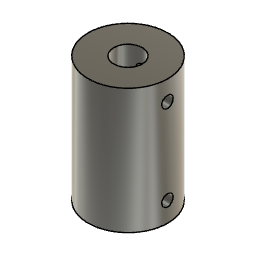
coupling (Autodesk Fusion 360 design; units mm, degrees)
Autodesk Fusion 360 part; units mm, degrees
note: some values were not read from the file. Set by a fixed rule: which sketch regions a step uses.
sketch "スケッチ1" plane through (0, 0, 0) normal (0, 0, 1) x (1, 0, 0)
  circle A0 centre (0, 0) radius 7
  dimension "d1" = 14
  constraint coincident A0.centre origin
  measures "d1" diameter of A0
extrude "押し出し1" add sketch "スケッチ1" along normal blind 12
extrude "押し出し2" add 1 faces at (1.11, -1.8763, 12) along direction (0, 0, 1) blind 10
sketch "スケッチ2" plane through (0, 0, 22) normal (0, 0, 1) x (-1, 0, 0)
  circle A0 centre (0, 0) radius 7
  circle A1 centre (0, 0) radius 2.5
  dimension "d6" = 5
  constraint coincident A0.centre A1.centre
  measures "d6" diameter of A1
sketch "スケッチ3" plane through (0, 0, 0) normal (0, 0, -1) x (1, 0, 0)
  circle A0 centre (0, 0) radius 7
  circle A1 centre (0, 0) radius 1.5
  dimension "d7" = 3
  constraint coincident A0.centre A1.centre
  measures "d7" diameter of A1
extrude "押し出し3" cut sketch "スケッチ3" against normal blind 11 contours A1
extrude "押し出し4" cut sketch "スケッチ2" against normal blind 11 contours A1
sketch "スケッチ4" plane through (0, 0, 0) normal (0, 1, 0) x (1, 0, 0)
  line L0 (-7, -22) -> (7, -22)
  line L1 (7, -22) -> (7, 0)
  line L2 (7, 0) -> (-7, 0)
  line L3 (-7, 0) -> (-7, -22)
  line L4 (-7, -22) -> (-7, -18.5)
  line L5 (-7, -18.5) -> (7, -18.5)
  line L6 (7, -22) -> (7, -18.5)
  line L7 (0, -22) -> (0, 0)
  circle A0 centre (0, -18.5) radius 1
  line L8 (-7, 0) -> (-7, -3.5)
  line L9 (-7, -3.5) -> (7, -3.5)
  circle A1 centre (0, -3.5) radius 1
  dimension "d12" = 3.5
  dimension "d13" = 2
  dimension "d20" = 3.5
  dimension "d21" = 2
  constraint horizontal L0
  constraint vertical L1
  constraint horizontal L2
  constraint vertical L3
  constraint perpendicular L0 L4
  constraint coincident L1 L5.end
  constraint perpendicular L1 L5
  constraint midpoint L0 L7.start
  constraint coincident L7.end origin
  constraint perpendicular L2 L7
  constraint midpoint L5 A0.centre
  constraint perpendicular L2 L8
  constraint coincident L1 L9.end
  constraint perpendicular L1 L9
  constraint midpoint L9 A1.centre
  measures "d12" distance of L0.start L4.end
  measures "d13" diameter of A0
  measures "d20" distance of L2.end L8.end
  measures "d21" diameter of A1
extrude "押し出し5" cut sketch "スケッチ4" along normal blind 10 contours L5 L7 A0 | L5 L7 A0 | L5 L7 A0 | L5 L7 A0
sketch "スケッチ5" plane through (0, 0, 0) normal (1, 0, 0) x (0, 1, 0)
  line L0 (-7, 22) -> (7, 22)
  line L1 (7, 22) -> (7, 0)
  line L2 (7, 0) -> (-7, 0)
  line L3 (-7, 0) -> (-7, 22)
  line L4 (-7, 22) -> (-7, 18.5)
  line L5 (-7, 22) -> (7, 22)
  line L6 (7, 22) -> (7, 18.5)
  line L7 (7, 18.5) -> (-7, 18.5)
  line L8 (-7, 18.5) -> (-7, 22)
  circle A0 centre (0, 18.5) radius 1
  line L9 (7, 0) -> (7, 3.5)
  line L10 (7, 3.5) -> (-7, 3.5)
  circle A1 centre (0, 3.5) radius 1
  dimension "d16" = 3.5
  dimension "d17" = 2
  dimension "d24" = 3.5
  dimension "d25" = 2
  constraint horizontal L0
  constraint vertical L1
  constraint horizontal L2
  constraint vertical L3
  constraint perpendicular L0 L4
  constraint horizontal L5
  constraint vertical L6
  constraint horizontal L7
  constraint vertical L8
  constraint coincident L1 L6.end
  constraint midpoint L7 A0.centre
  constraint perpendicular L2 L9
  constraint coincident L3 L10.end
  constraint perpendicular L3 L10
  constraint midpoint L10 A1.centre
  measures "d16" distance of L0.start L4.end
  measures "d17" diameter of A0
  measures "d24" distance of L1.end L9.end
  measures "d25" diameter of A1
extrude "押し出し6" cut sketch "スケッチ5" along normal blind 10 contours L7 A0 | L7 A0
extrude "押し出し7" cut sketch "スケッチ4" along normal blind 10 contours L7 L9 A1 | L7 L9 A1 | L7 L9 A1 | L7 L9 A1
extrude "押し出し8" cut sketch "スケッチ5" along normal blind 10 contours L10 A1 | L10 A1
